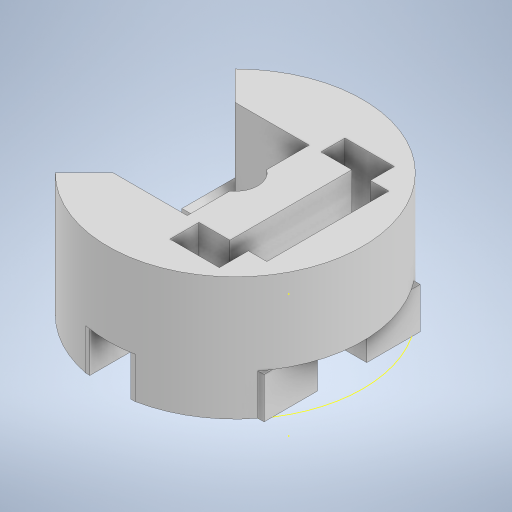
# Autodesk Inventor part: ServoUtmater1
Saved by Autodesk Inventor 2023 (Build 270158000, 158)
## iProperties
Created: 2023-04-11
Part Number: ServoUtmater1
Material: Generic
Document SubType Name: Modeling
Designer: Anders
Density: 1 g/cm^3
Appearance: Default
Author: Anders
## iProperties of the stored document ServoUtmater_3DPrint.ipt
Created: 2023-04-11
Part Number: ServoUtmater_3DPrint
Material: Generic
Document SubType Name: Modeling
Designer: Anders
Density: 1 g/cm^3
Appearance: Default
Author: Anders
Autodesk Inventor part; units mm, degrees
ref_plane "YZ Plane" through (0, 0, 0) normal (1, 0, 0) x (0, 1, 0)
ref_plane "XZ Plane" through (0, 0, 0) normal (0, 1, 0) x (-1, 0, 0)
ref_plane "XY Plane" through (0, 0, 0) normal (0, 0, 1) x (1, 0, 0)
sketch "Sketch5" plane through (0, 0, 0) normal (0, 1, 0) x (-1, 0, 0)
  line L0 (0, 0) -> (32, 0)
  line L1 (32, 0) -> (32, -19)
  line L2 (32, -19) -> (0, -19)
  line L3 (0, -19) -> (0, 0)
  line L4 (32, -19) -> (19, -19)
  line L5 (19, -19) -> (19, 0)
  line L6 (19, 0) -> (32, 0)
  line L7 (32, 0) -> (32, -19)
  line L8 (0, 0) -> (13, 0)
  line L9 (13, 0) -> (13, -19)
  line L10 (13, -19) -> (0, -19)
  line L11 (0, -19) -> (0, 0)
  line L12 (0, 0) -> (32, 0)
  line L13 (32, 0) -> (32, -6.75)
  line L14 (32, -6.75) -> (0, -6.75)
  line L15 (0, -6.75) -> (0, 0)
  line L16 (0, -19) -> (32, -19)
  line L17 (32, -19) -> (32, -12.25)
  line L18 (32, -12.25) -> (0, -12.25)
  line L19 (0, -12.25) -> (0, -19)
  circle A0 centre (16, -9.5) radius 4
  circle A1 centre (16, -9.5) radius 1
  line L20 (13, 0) -> (19, 0)
  line L21 (19, 0) -> (19, -19)
  line L22 (19, -19) -> (13, -19)
  line L23 (13, -19) -> (13, 0)
  point P0 (13, -12.1458)
  point P1 (13.0953, -12.25)
  point P2 (0, -12.25)
  point P3 (13, -19)
  point P4 (13.0953, -6.75)
  point P5 (13, -6.8542)
  point P6 (19, -6.8542)
  point P7 (18.9047, -6.75)
  point P8 (19, 0)
  point P9 (18.9047, -12.25)
  point P10 (19, -12.1458)
  point P11 (13, -12.25)
  point P12 (13, -6.75)
  point P13 (19, -6.75)
  point P14 (19, -12.25)
  dimension "d13" = 32
  dimension "d14" = 19
  dimension "d15" = 13
  dimension "d16" = 19
  dimension "d17" = 13
  dimension "d18" = 19
  dimension "d19" = 32
  dimension "d20" = 6.75
  dimension "d21" = 32
  dimension "d22" = 6.75
  dimension "d23" = 8
  dimension "d24" = 2
  constraints: 48 end point, 12 parallel, 6 horizontal, 6 perpendicular, 2 centre point, 1 coincident
  measures "d13" distance of L1.end L2.end
  measures "d14" distance of L0.end L1.end
  measures "d15" distance of L5.end L6.end
  measures "d16" distance of L4.end L5.end
  measures "d17" distance of L9.end L10.end
  measures "d18" distance of L8.end L9.end
  measures "d19" distance of L13.end L14.end
  measures "d20" distance of L12.end L13.end
  measures "d21" distance of L18.end L17.end
  measures "d22" distance of L17.end L16.end
  measures "d23" diameter of A0
  measures "d24" diameter of A1
extrude "Extrusion2" add sketch "Sketch5" along normal blind 5 contours L0 L9 L14 L3 | L0 L5 L14 A0 L9 | L14 L9 A0 L18 L3 | L0 L1 L14 L5 | L14 A0 L9 | L18 L9 L2 L3 | L14 L1 L18 L5 A0 | L5 A0 L14 | L9 A0 | A0 L14 | L18 A0 L5 L2 L9 | L9 A0 L18 | A0 L5 | L18 A0 | L1 L2 L5 L18 | L5 L18 A0
sketch "Sketch6" plane through (0, 5, 0) normal (0, 1, 0) x (1, 0, 0)
  arc A0 (-18.9047, 6.75) -> (-19, 6.8542) centre (-16, 9.5) ccw projected
  circle A1 centre (-16, 9.5) radius 15.5
  line L0 (-16, 9.5) -> (-26.9602, 20.4602)
  line L1 (-16, 9.5) -> (-0.5, 9.5) construction
  line L2 (-16, 9.5) -> (-26.9602, -1.4602)
  line L3 (-16, 9.5) -> (-0.5, 9.5) construction
  line L4 (-26.9602, -1.4602) -> (-19.8891, 5.6109)
  line L5 (-19.8891, 5.6109) -> (-19.8891, 13.3891)
  circle A2 centre (-16, 9.5) radius 1
  point P0 (0, 0)
  dimension "d27" = 31
  dimension "d28" = 135
  dimension "d29" = 135
  dimension "d30" = 10
  dimension "d33" = 2
  constraints: 12 end point, 2 centre point, 2 coincident, 2 equal length, 2 horizontal, 2 point on circle, 2 point on line, 1 vertical
  measures "d27" diameter of A1
  measures "d28" angle of L1 L0
  measures "d29" angle of L2 L3
  measures "d30" distance of L2.end L4.end
  measures "d33" diameter of A2
extrude "Extrusion3" add sketch "Sketch6" along normal blind 10 contours L2 A2 L0 A0 | L2 L5 A0 L0 A2 | A0 L0 A1 L2 | A0 L5 L0
sketch "Sketch7" plane through (0, 15, 0) normal (0, 1, 0) x (1, 0, 0)
  circle A0 centre (-16, 9.5) radius 1 projected
  circle A1 centre (-16, 9.5) radius 2.75
  point P0 (0, 0)
  dimension "d34" = 5.5
  constraints: 1 centre point, 1 coincident
  measures "d34" diameter of A1
extrude "Extrusion4" cut sketch "Sketch7" against normal blind 10
sketch "Sketch8" plane through (0, 0, 0) normal (0, -1, 0) x (1, 0, 0)
  point P0 (0, 0)
sketch "Sketch9" plane through (0, 0, 0) normal (0, -1, 0) x (1, 0, 0)
  arc A0 (-3.7526, -19) -> (-3.7526, 0) centre (-16, -9.5) ccw projected
  point P0 (0, 0)
sketch "Sketch10" plane through (0, 0, 0) normal (0, -1, 0) x (1, 0, 0)
  line L0 (-32, 0) -> (-25.5, 0) projected
  line L1 (-32, 0) -> (-19, 0)
  line L2 (-19, 0) -> (-19, -6)
  line L3 (-19, -6) -> (-32, -6)
  line L4 (-32, -6) -> (-32, 0)
  line L5 (-32, -19) -> (-32, 0) projected
  line L6 (-32, -19) -> (-19, -19)
  line L7 (-19, -19) -> (-19, -13)
  line L8 (-19, -13) -> (-32, -13)
  line L9 (-32, -13) -> (-32, -19)
  line L10 (0, 0) -> (-13, 0)
  line L11 (-13, 0) -> (-13, -6)
  line L12 (-13, -6) -> (0, -6)
  line L13 (0, -6) -> (0, 0)
  line L14 (0, -19) -> (-3.7526, -19) projected
  line L15 (0, -19) -> (-13, -19)
  line L16 (-13, -19) -> (-13, -13)
  line L17 (-13, -13) -> (0, -13)
  line L18 (0, -13) -> (0, -19)
  line L19 (-19, -6) -> (-13, -6)
  line L20 (-13, -6) -> (-13, -13)
  line L21 (-13, -13) -> (-19, -13)
  line L22 (-19, -13) -> (-19, -6)
  line L23 (-19, 0) -> (-13, 0)
  line L24 (-13, 0) -> (-13, -6)
  line L25 (-13, -6) -> (-19, -6)
  line L26 (-19, -6) -> (-19, 0)
  line L27 (-13, -13) -> (-19, -13)
  line L28 (-19, -13) -> (-19, -19)
  line L29 (-19, -19) -> (-13, -19)
  line L30 (-13, -19) -> (-13, -13)
  line L31 (-32, -13) -> (-19, -13)
  line L32 (-19, -13) -> (-19, -6)
  line L33 (-19, -6) -> (-32, -6)
  line L34 (-32, -6) -> (-32, -13)
  line L35 (-13, -6) -> (0, -6)
  line L36 (0, -6) -> (0, -13)
  line L37 (0, -13) -> (-13, -13)
  line L38 (-13, -13) -> (-13, -6)
  point P0 (0, -6)
  dimension "d37" = 13
  dimension "d38" = 6
  dimension "d39" = 6
  dimension "d40" = 13
  dimension "d41" = 6
  dimension "d42" = 13
  dimension "d43" = 6
  constraints: 72 end point, 18 parallel, 9 horizontal, 9 perpendicular
  measures "d37" distance of L2.end L3.end
  measures "d38" distance of L1.end L2.end
  measures "d39" distance of L7.end L6.end
  measures "d40" distance of L12.end L11.end
  measures "d41" distance of L11.end L10.end
  measures "d42" distance of L16.end L17.end
  measures "d43" distance of L15.end L16.end
extrude "Extrusion5" cut sketch "Sketch10" against normal blind 5 contours L3 L22 L8 L5 | L23 L11 L19 L2 | L19 L20 L21 L22 | L12 L36 L17 L20 | L21 L16 L29 L7
sketch "Sketch11" plane through (0, 5, 0) normal (0, -1, 0) x (1, 0, 0)
  arc A0 (-3.7526, 0) -> (-26.9602, 1.4602) centre (-16, -9.5) ccw projected
  arc A1 (-26.9602, -20.4602) -> (-3.7526, -19) centre (-16, -9.5) ccw projected
  line L0 (-25.5, 0) -> (-26.9602, 1.4602) projected
  line L1 (-26.9602, -20.4602) -> (-25.5, -19) projected
  line L2 (-13, 0) -> (-3.7526, 0) projected
  line L3 (-19, -13) -> (-19.8891, -13) projected
  line L4 (-13, -13) -> (-13, -19) projected
  line L5 (-25.5, 0) -> (-19, 0) projected
  line L6 (-25.5, 0) -> (-3.7526, 0)
  line L7 (-19, -19) -> (-32, -19) projected
  line L8 (-19, -19) -> (-19, -13) projected
  line L9 (0, -19) -> (-13, -19) projected
  line L10 (-13, -13) -> (-13, -19) projected
  line L11 (-19.8891, -13.3891) -> (-25.5, -19) projected
  line L12 (-25.5, -19) -> (-3.7526, -19)
  line L13 (-19, 0) -> (-13, 0)
  line L14 (-13, 0) -> (-13, 7)
  line L15 (-13, 7) -> (-19, 7)
  line L16 (-19, 7) -> (-19, 0)
  line L17 (-19, -13) -> (-13, -13)
  line L18 (-13, -13) -> (-13, -25.2796)
  line L19 (-13, -25.2796) -> (-19, -25.2796)
  line L20 (-19, -25.2796) -> (-19, -13)
  point P0 (0, 0)
  point P1 (-19, -24.7069)
  point P2 (-13, -24.7069)
  point P3 (-13, 5.7069)
  point P4 (-19, 5.7069)
  dimension "d47" = 7
  constraints: 20 end point, 4 parallel, 3 horizontal, 2 perpendicular, 1 point on line
  measures "d47" distance of L14.end L13.end
extrude "Extrusion6" add sketch "Sketch11" along normal blind 5 contours L2 L14 A0 | L16 L5 L0 A0 | L1 L7 L20 A1 | L18 L9 A1
sketch "Sketch12" plane through (0, 15, 0) normal (0, 1, 0) x (1, 0, 0)
  point P0 (0, 0)
sketch "Sketch14" plane through (0, 0, 0) normal (1, 0, 0) x (0, 0, -1)
  line L0 (0, 5) -> (6, 5) projected
  line L1 (6, 0) -> (6, 5) projected
  line L2 (0, 0) -> (6, 0) projected
  line L3 (0, 0) -> (0, 5) projected
  line L4 (13, 5) -> (13, 0) projected
  line L5 (13, 0) -> (19, 0) projected
  line L6 (19, 0) -> (19, 5) projected
  line L7 (13, 5) -> (19, 5) projected
  line L8 (-5.7069, 0) -> (6, 0) projected
  line L9 (0, 5) -> (6, 5)
  line L10 (6, 5) -> (6, 0)
  line L11 (6, 0) -> (0, 0)
  line L12 (0, 0) -> (0, 5)
  line L13 (13, 0) -> (24.7069, 0) projected
  line L14 (13, 0) -> (19, 0)
  line L15 (19, 0) -> (19, 5)
  line L16 (19, 5) -> (13, 5)
  line L17 (13, 5) -> (13, 0)
  constraints: 16 end point, 4 parallel, 2 horizontal, 2 perpendicular
extrude "Extrusion8" cut sketch "Sketch14" against normal blind 3
sketch "Sketch16" plane through (-32, 0, -19) normal (-1, 0, 0) x (0, 0, 1)
  line L0 (0, 5) -> (6, 5) projected
  line L1 (0, 0) -> (0, 5) projected
  line L2 (0, 0) -> (6, 0) projected
  line L3 (6, 0) -> (6, 5) projected
  line L4 (13, 0) -> (19, 0) projected
  line L5 (13, 5) -> (13, 0) projected
  line L6 (13, 5) -> (19, 5) projected
  line L7 (19, 0) -> (19, 5) projected
  line L8 (0, 5) -> (0, 0) projected
  line L9 (6, 0) -> (6, 5) projected
  line L10 (0, 5) -> (6, 5)
  line L11 (6, 5) -> (6, 0)
  line L12 (6, 0) -> (0, 0)
  line L13 (0, 0) -> (0, 5)
  line L14 (13, 0) -> (13, 5) projected
  line L15 (19, 0) -> (19, 5) projected
  line L16 (13, 0) -> (19, 0)
  line L17 (19, 0) -> (19, 5)
  line L18 (19, 5) -> (13, 5)
  line L19 (13, 5) -> (13, 0)
  constraints: 16 end point, 4 parallel, 2 horizontal, 2 perpendicular
extrude "Extrusion9" cut sketch "Sketch16" against normal blind 6.5
sketch "Sketch18" plane through (0, 15, 0) normal (0, 1, 0) x (1, 0, 0)
  line L0 (-19.8891, 5.6109) -> (-26.9602, -1.4602) projected
  line L1 (-26.9602, 20.4602) -> (-19.8891, 13.3891) projected
  line L2 (-23.4246, 2.0754) -> (-14.4246, 2.0754)
  line L3 (-14.4246, 2.0754) -> (-14.4246, 16.9246)
  line L4 (-14.4246, 16.9246) -> (-23.4246, 16.9246)
  line L5 (-23.4246, 16.9246) -> (-23.4246, 2.0754)
  line L6 (-9.2348, 2.0754) -> (-4.7348, 2.0754)
  line L7 (-4.7348, 2.0754) -> (-4.7348, 16.9246)
  line L8 (-4.7348, 16.9246) -> (-9.2348, 16.9246)
  line L9 (-9.2348, 16.9246) -> (-9.2348, 2.0754)
  line L10 (-13, 6) -> (-13, -5.7069) projected
  line L11 (-6.9848, -1.4602) -> (-13, -1.4602)
  line L12 (-13, -1.4602) -> (-13, 2.0754)
  line L13 (-13, 2.0754) -> (-6.9848, 2.0754)
  line L14 (-6.9848, 2.0754) -> (-6.9848, -1.4602)
  line L15 (-13, 13) -> (-13, 24.7069) projected
  line L16 (-6.9848, 19.8513) -> (-13, 19.8513)
  line L17 (-13, 19.8513) -> (-13, 16.9246)
  line L18 (-13, 16.9246) -> (-6.9848, 16.9246)
  line L19 (-6.9848, 16.9246) -> (-6.9848, 19.8513)
  point P0 (0, 0)
  dimension "d79" = 9
  dimension "d80" = 4.5
  constraints: 32 end point, 8 parallel, 5 point on line, 4 horizontal, 4 perpendicular, 1 midpoint
  measures "d79" distance of L4.end L3.end
  measures "d80" distance of L8.end L7.end
extrude "Extrusion12" cut sketch "Sketch18" against normal blind 10
sketch "Sketch19" plane through (-13, 0, -6) normal (-1, 0, 0) x (0, 0, 1)
  line L0 (11.7069, 5) -> (11.7069, 0) projected
  line L1 (11.7069, 0) -> (0, 0) projected
  line L2 (11.7069, 5) -> (0, 5)
  line L3 (0, 5) -> (0, 0)
  line L4 (0, 0) -> (11.7069, 0)
  line L5 (11.7069, 0) -> (11.7069, 5)
  line L6 (-7, 0) -> (-7, 5) projected
  line L7 (-7, 0) -> (-18.7069, 0) projected
  line L8 (-18.7069, 5) -> (-18.7069, 0) projected
  line L9 (-7, 5) -> (-10.9246, 5) projected
  line L10 (-7, 5) -> (-18.7069, 5)
  line L11 (-18.7069, 5) -> (-18.7069, 0)
  line L12 (-18.7069, 0) -> (-7, 0)
  line L13 (-7, 0) -> (-7, 5)
  point P0 (6, 0)
  constraints: 16 end point, 4 parallel, 2 horizontal, 2 perpendicular
sketch "Sketch20" plane through (-19, 0, 5.7069) normal (1, 0, 0) x (0, 0, -1)
  line L0 (11.7069, 0) -> (0, 0) projected
  line L1 (11.7069, 0) -> (11.7069, 5) projected
  line L2 (0, 0) -> (11.7069, 0)
  line L3 (11.7069, 0) -> (11.7069, 5)
  line L4 (11.7069, 5) -> (0, 5)
  line L5 (0, 5) -> (0, 0)
  line L6 (18.7069, 0) -> (18.7069, 5) projected
  line L7 (22.6315, 5) -> (30.4138, 5) projected
  line L8 (18.7069, 0) -> (30.4138, 0)
  line L9 (30.4138, 0) -> (30.4138, 5)
  line L10 (30.4138, 5) -> (18.7069, 5)
  line L11 (18.7069, 5) -> (18.7069, 0)
  point P0 (5.7069, 0)
  point P1 (18.7069, 5)
  constraints: 16 end point, 4 parallel, 2 horizontal, 2 perpendicular
extrude "Extrusion13" add sketch "Sketch19" along normal blind 0.5
extrude "Extrusion14" add sketch "Sketch20" along normal blind 0.5
sketch "Sketch23" plane through (-3, 0, -13) normal (0, 0, 1) x (1, 0, 0)
  line L0 (0, 5) -> (-1.7348, 5) projected
  line L1 (0, 5) -> (-10.5, 5)
  line L2 (-10.5, 5) -> (-10.5, 0)
  line L3 (-10.5, 0) -> (0, 0)
  line L4 (0, 0) -> (0, 5)
  line L5 (-15.5, 0) -> (-22.5, 0) projected
  line L6 (-22.5, 5) -> (-22.5, 0) projected
  line L7 (-15.5, 0) -> (-22.5, 0)
  line L8 (-22.5, 0) -> (-22.5, 5)
  line L9 (-22.5, 5) -> (-15.5, 5)
  line L10 (-15.5, 5) -> (-15.5, 0)
  point P0 (3, 0)
  constraints: 16 end point, 4 parallel, 2 horizontal, 2 perpendicular
sketch "Sketch24" plane through (-3, 0, -6) normal (0, 0, -1) x (-1, 0, 0)
  line L0 (0, 0) -> (0, 5) projected
  line L1 (10.5, 5) -> (6.2348, 5) projected
  line L2 (0, 0) -> (10.5, 0)
  line L3 (10.5, 0) -> (10.5, 5)
  line L4 (10.5, 5) -> (0, 5)
  line L5 (0, 5) -> (0, 0)
  line L6 (22.5, 5) -> (15.5, 5) projected
  line L7 (22.5, 0) -> (22.5, 5) projected
  line L8 (15.5, 5) -> (22.5, 5)
  line L9 (22.5, 5) -> (22.5, 0)
  line L10 (22.5, 0) -> (15.5, 0)
  line L11 (15.5, 0) -> (15.5, 5)
  point P0 (-3, 0)
  constraints: 16 end point, 4 parallel, 2 horizontal, 2 perpendicular
extrude "Extrusion15" add sketch "Sketch24" along normal blind 0.5
extrude "Extrusion16" add sketch "Sketch23" along normal blind 0.5
body "Solid2"
